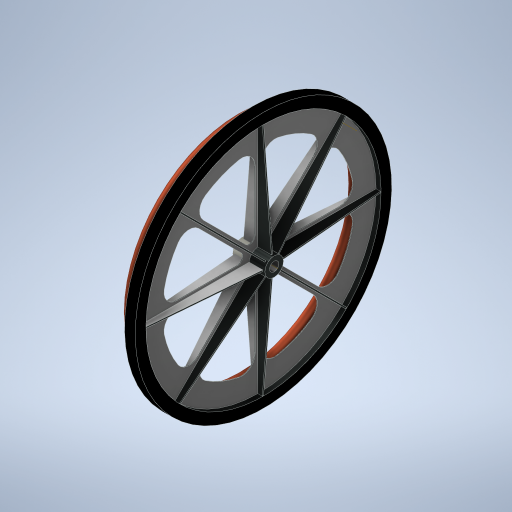
# Autodesk Inventor part: Rear wheel
Saved by Autodesk Inventor 2023 (Build 270158000, 158)
## iProperties
Created: 2023-10-30
Part Number: Rear wheel
Material: Generic
Document SubType Name: Modeling
Designer: Raghav
Density: 1 g/cm^3
Appearance: Gunmetal - Polished
Author: Raghav
Autodesk Inventor part; units mm, degrees
ref_plane "YZ Plane" through (0, 0, 0) normal (1, 0, 0) x (0, 1, 0)
sketch "Sketch1" plane through (0, 0, 0) normal (1, 0, 0) x (0, 1, 0)
  circle A0 centre (0, 0) radius 22.225
  dimension "d0" = 44.45
  constraints: 1 centre point, 1 coincident
  measures "d0" diameter of A0
extrude "Extrusion1" add sketch "Sketch1" along normal blind 38.1 and the other way blind 38.1
sketch "Sketch2" plane through (0, 0, 0) normal (1, 0, 0) x (0, 1, 0)
  circle A0 centre (0, 0) radius 304.8
  dimension "d5" = 609.6
  constraints: 1 centre point, 1 coincident
  measures "d5" diameter of A0
extrude "Extrusion2" add sketch "Sketch2" along normal blind 0.762 and the other way blind 0.762
sketch "Sketch3" plane through (0, 0, 0) normal (1, 0, 0) x (0, 1, 0)
  circle A0 centre (0, 0) radius 304.8 projected
  circle A1 centre (0, 0) radius 279.4
  dimension "d10" = 25.4
  constraints: 1 centre point
  measures "d10" radial gap between concentric circles of A0 A1
extrude "Extrusion3" add sketch "Sketch3" along normal blind 12.7 and the other way blind 12.7
sketch "Sketch4" plane through (0.762, 0, 0) normal (1, 0, 0) x (0, 0, -1)
  line L0 (0, 0) -> (0, 279.4)
  circle A0 centre (0, 0) radius 279.4 projected
  line L1 (0, 0) -> (197.5656, 197.5656)
  arc A1 (125.7356, 190.9149) -> (46.0887, 223.9058) centre (0, 0) ccw
  line L2 (7.9375, 192.8077) -> (7.9375, 49.8233)
  arc A2 (7.9375, 49.8233) -> (29.6178, 40.8431) centre (20.6375, 49.8233) ccw
  line L3 (29.6178, 40.8431) -> (130.723, 141.9483)
  arc A3 (130.723, 141.9483) -> (125.7356, 190.9149) centre (108.2724, 164.399) ccw
  arc A4 (46.0887, 223.9058) -> (7.9375, 192.8077) centre (39.6875, 192.8077) ccw
  dimension "d15" = 45
  dimension "d16" = 50.8
  dimension "d17" = 15.875
  dimension "d18" = 15.875
  dimension "d19" = 12.7
  dimension "d20" = 31.75
  constraints: 10 point on circle, 8 end point, 6 tangent, 4 centre point, 2 parallel, 2 vertical, 1 equal radius
  measures "d15" angle of L1 L0
  measures "d16" radial gap between concentric circles of A0 A1
  measures "d17" diameter of L2 L0
  measures "d18" diameter of L3 L1
  measures "d19" radius of A2
  measures "d20" radius of A3
extrude "Extrusion4" cut sketch "Sketch4" against normal blind 165.1 contours A3 L3 A2 L2 A4 A1
ref_plane "Work Plane1" through (0, 281.94, 0) normal (0, 1, 0) x (-1, 0, 0)
sketch "Sketch5" plane through (0, 0, 0) normal (0, 1, 0) x (-1, 0, 0)
  line L0 (-34.925, 1.5875) -> (34.925, 1.5875)
  line L1 (34.925, 1.5875) -> (34.925, -1.5875)
  line L2 (34.925, -1.5875) -> (-34.925, -1.5875)
  line L3 (-34.925, -1.5875) -> (-34.925, 1.5875)
  line L4 (-34.925, 1.5875) -> (34.925, -1.5875) construction
  line L5 (34.925, 1.5875) -> (-34.925, -1.5875) construction
  line L6 (38.1, -22.225) -> (38.1, 22.225) projected
  point P0 (0, 0)
  dimension "d24" = 3.175
  dimension "d25" = 3.175
  constraints: 12 end point, 2 midpoint, 2 parallel, 1 horizontal, 1 perpendicular
  measures "d24" distance between parallel lines of L6 L1
  measures "d25" distance of L2.end L0.start
sketch "Sketch6" plane through (0, 281.94, 0) normal (0, 1, 0) x (-1, 0, 0)
  line L0 (-11.1125, 1.5875) -> (11.1125, 1.5875)
  line L1 (11.1125, 1.5875) -> (11.1125, -1.5875)
  line L2 (11.1125, -1.5875) -> (-11.1125, -1.5875)
  line L3 (-11.1125, -1.5875) -> (-11.1125, 1.5875)
  line L4 (-11.1125, 1.5875) -> (11.1125, -1.5875) construction
  line L5 (11.1125, 1.5875) -> (-11.1125, -1.5875) construction
  point P0 (0, 0)
  dimension "d26" = 22.225
  dimension "d27" = 3.175
  constraints: 12 end point, 2 midpoint, 2 parallel, 1 horizontal, 1 perpendicular
  measures "d26" distance of L1.end L2.end
  measures "d27" distance of L0.end L1.end
loft "Loft1" add profiles "Sketch5", "Sketch6"
sketch "Sketch7" plane through (-0.762, 0, 0) normal (-1, 0, 0) x (0, 0, 1)
  circle A0 centre (0, 266.7) radius 5.5565
  point P0 (0, 0)
  dimension "d32" = 11.113
  dimension "d33" = 266.7
  constraints: 1 centre point
  measures "d32" diameter of A0
  measures "d33" distance of point (0, 0) A0.centre
extrude "Extrusion5" add sketch "Sketch7" along normal blind 28.575
pattern_circular "Circular Pattern1" count 8 over 360 about axis through (-38.1, 0, 0) along (-1, 0, 0) of "Loft1", "Extrusion5", "Extrusion4"
sketch "Sketch8" plane through (-38.1, 0, 0) normal (-1, 0, 0) x (0, 0, 1)
  circle A0 centre (0, 0) radius 11.1125
  dimension "d39" = 22.225
  constraints: 1 centre point, 1 coincident
  measures "d39" diameter of A0
extrude "Extrusion6" cut sketch "Sketch8" against normal blind 357.1875
ref_plane "Work Plane2" through (-29.337, 188.5854, -188.5854) normal (0, -0.7071, -0.7071) x (-1, 0, 0)
sketch "Sketch9" plane through (-29.337, 188.5854, -188.5854) normal (0, -0.7071, -0.7071) x (-1, 0, 0)
  circle A0 centre (9.525, 0) radius 9.525
  line L0 (0, -5.5565) -> (0, 5.5565) construction
  line L1 (0, 5.5565) -> (0, -5.5565)
  point P0 (-29.337, -266.7)
  dimension "d42" = 19.05
  constraints: 2 end point, 1 centre point, 1 collinear, 1 tangent
  measures "d42" diameter of A0
sketch "Sketch10" plane through (-29.337, 188.5854, -188.5854) normal (0, -0.7071, -0.7071) x (-1, 0, 0)
  line L0 (-29.337, -266.7) -> (61.9125, -266.7)
  constraints: 2 end point, 1 horizontal
revolve "Revolution1" add sketch "Sketch9" angle 360 about axis through (0, 0, 0) along (-1, 0, 0)
body "Solid1"
